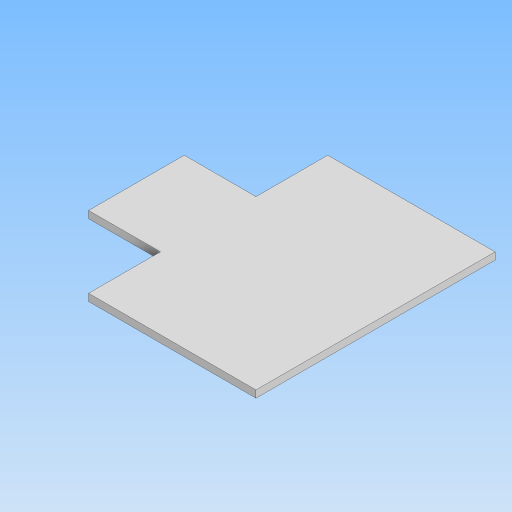
# Autodesk Inventor part: Ploschka
Saved by Autodesk Inventor 2023 (Build 270158000, 158)
## iProperties
Created: 2023-08-09
Part Number: Ploschka
Material: Generic
Document SubType Name: Modeling
Designer: MenMe
Density: 1 g/cm^3
Appearance: Default
Author: MenMe
Autodesk Inventor part; units mm, degrees
ref_plane "YZ Plane" through (0, 0, 0) normal (1, 0, 0) x (0, 1, 0)
ref_plane "XZ Plane" through (0, 0, 0) normal (0, 1, 0) x (-1, 0, 0)
ref_plane "XY Plane" through (0, 0, 0) normal (0, 0, 1) x (1, 0, 0)
sketch "Sketch1" plane through (0, 0, 0) normal (0, 1, 0) x (-1, 0, 0)
  line L0 (0, 0) -> (0, -100)
  line L1 (0, -100) -> (70, -100)
  line L2 (70, -100) -> (70, -70)
  line L3 (70, -70) -> (100, -70)
  line L4 (100, -70) -> (100, -30)
  line L5 (100, -30) -> (70, -30)
  line L6 (70, -30) -> (70, 0)
  line L7 (70, 0) -> (0, 0)
  dimension "d0" = 100
  dimension "d1" = 70
  dimension "d3" = 30
  dimension "d4" = 30
  dimension "d5" = 70
  dimension "d6" = 30
  constraints: 16 end point, 6 perpendicular, 2 vertical
  measures "d0" distance of L0.start L0.end
  measures "d1" distance of L6.end L0.start
  measures "d3" distance of L5.end L6.end
  measures "d4" distance of L2.end L1.end
  measures "d5" distance of L0.end L1.end
  measures "d6" distance of L2.end L3.end
extrude "Extrusion1" add sketch "Sketch1" along normal blind 3
body "Solid1"
